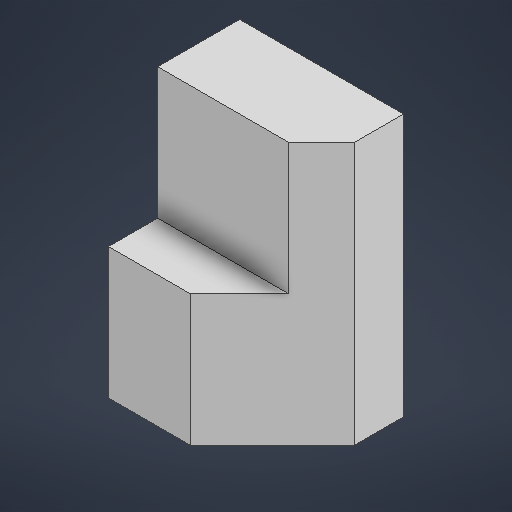
# Autodesk Inventor part: Peça2
Saved by Autodesk Inventor 2027.1 (Build 311270010, 270A)
## iProperties
Created: 2026-09-24
Part Number: Peça2
Material: Genérico
Document SubType Name: Modeling
Designer: carlo
Density: 1 g/cm^3
Appearance: Padrão
Author: carlo
Autodesk Inventor part; units mm, degrees
ref_plane "YZ Plane" through (0, 0, 0) normal (1, 0, 0) x (0, 1, 0)
ref_plane "XZ Plane" through (0, 0, 0) normal (0, 1, 0) x (-1, 0, 0)
ref_plane "XY Plane" through (0, 0, 0) normal (0, 0, 1) x (1, 0, 0)
sketch "Esboço1" plane through (0, 0, 0) normal (0, 1, 0) x (-1, 0, 0)
  line L0 (-25, 20) -> (25, 20)
  line L1 (25, 20) -> (25, -20)
  line L2 (25, -20) -> (-25, -20)
  line L3 (-25, -20) -> (-25, 20)
  line L4 (-25, 20) -> (25, -20) construction
  line L5 (25, 20) -> (-25, -20) construction
  point P0 (0, 0)
  dimension "d0" = 50
  dimension "d1" = 40
  constraints: 12 end point, 2 midpoint, 2 parallel, 1 horizontal, 1 perpendicular
  measures "d0" distance of L1.end L2.end
  measures "d1" distance of L0.end L1.end
extrude "Extrusão1" add sketch "Esboço1" along normal blind 80
chamfer "Chanfro1" distance 25 angle 45 1 edges at (25, 40, 20) measured on face at (-8.3333, 26.6667, 20)
sketch "Esboço2" plane through (-25, 0, -20) normal (-1, 0, 0) x (0, 0, 1)
  line L0 (0, 80) -> (40, 80) projected
  line L1 (40, 80) -> (25, 80)
  line L2 (25, 80) -> (25, 40)
  line L3 (25, 40) -> (40, 40)
  line L4 (40, 40) -> (40, 80)
  point P0 (20, 0)
  dimension "d7" = 15
  dimension "d8" = 40
  constraints: 8 end point, 2 parallel, 1 perpendicular, 1 point on line
  measures "d7" distance of L0.end L1.end
  measures "d8" distance of L2.end L1.end
extrude "Extrusão2" cut sketch "Esboço2" against normal blind 80
